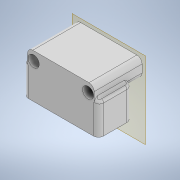
# Autodesk Inventor part: Кронштейн АКБ
Saved by Autodesk Inventor 2021 (Build 250183000, 183)
## iProperties
Created: 2023-02-18
Part Number: Кронштейн АКБ
Material: Типовые
Document SubType Name: Modeling
Designer: Tasya
Density: 1 g/cm^3
Appearance: По умолчанию
Author: Tasya
Autodesk Inventor part; units mm, degrees
ref_plane "YZ Plane" through (0, 0, 0) normal (1, 0, 0) x (0, 1, 0)
ref_plane "XZ Plane" through (0, 0, 0) normal (0, 1, 0) x (-1, 0, 0)
ref_plane "XY Plane" through (0, 0, 0) normal (0, 0, 1) x (1, 0, 0)
ref_plane "РабПлоскость1" through (0, 1, 4) normal (0, 0, 1) x (1, 0, 0)
sketch "Эскиз1" plane through (0, 1, 4) normal (0, 0, 1) x (1, 0, 0)
  circle A0 centre (-10.5, 2.5) radius 1.55 projected
  line L0 (12.85, -4) -> (12.85, 4) projected
  arc A1 (12.85, 4) -> (10.85, 6) centre (10.85, 4) ccw projected
  line L1 (10.85, 6) -> (-10.85, 6) projected
  arc A2 (-10.85, 6) -> (-12.85, 4) centre (-10.85, 4) ccw projected
  line L2 (-12.85, 4) -> (-12.85, -4) projected
  arc A3 (-12.85, -4) -> (-10.85, -6) centre (-10.85, -4) ccw construction
  line L3 (-10.85, -6) -> (-5, -6) construction
  line L4 (-3, -8) -> (-5, -6) construction
  line L5 (-3, -8) -> (-3, -21) construction
  line L6 (-3, -21) -> (3, -21) construction
  line L7 (3, -21) -> (3, -8) construction
  line L8 (5, -6) -> (3, -8) construction
  line L9 (5, -6) -> (10.85, -6) construction
  arc A4 (10.85, -6) -> (12.85, -4) centre (10.85, -4) ccw construction
  circle A5 centre (10.5, 2.5) radius 1.55 projected
  arc A6 (-12.85, 1) -> (-10.85, -1) centre (-10.85, 1) ccw projected
  line L10 (-10.85, -1) -> (10.85, -1) projected
  arc A7 (10.85, -1) -> (12.85, 1) centre (10.85, 1) ccw projected
  point P0 (0, -1)
extrude "Выдавливание1" add sketch "Эскиз1" along normal blind 18.5 contours A0 | A7 L10 A6 L2 A2 L1 A1 L0 | A5
sketch "Эскиз2" plane through (-10.85, 0, 4) normal (0, -1, 0) x (1, 0, 0)
  line L0 (10.85, -4) -> (10.85, 28) construction
  line L1 (23.35, 16.5) -> (-1.65, 16.5)
  line L2 (-1.65, 16.5) -> (-1.65, 7.5)
  line L3 (-1.65, 7.5) -> (23.35, 7.5)
  line L4 (23.35, 7.5) -> (23.35, 16.5)
  line L5 (23.35, 16.5) -> (-1.65, 7.5) construction
  line L6 (-1.65, 16.5) -> (23.35, 7.5) construction
  line L7 (-3.65, 7.5) -> (-3.65, 16.5)
  line L8 (-1.65, 18.5) -> (23.35, 18.5)
  line L9 (25.35, 16.5) -> (25.35, 7.5)
  line L10 (23.35, 5.5) -> (-1.65, 5.5)
  arc A0 (-3.65, 7.5) -> (-1.65, 5.5) centre (-1.65, 7.5) ccw
  arc A1 (-1.65, 18.5) -> (-3.65, 16.5) centre (-1.65, 16.5) ccw
  arc A2 (25.35, 16.5) -> (23.35, 18.5) centre (23.35, 16.5) ccw
  arc A3 (23.35, 5.5) -> (25.35, 7.5) centre (23.35, 7.5) ccw
  point P0 (10.85, 12)
  dimension "d2" = 25
  dimension "d3" = 9
  dimension "d4" = 16
  dimension "d5" = 2
  dimension "d6" = 2
  constraints: 22 end point, 8 point on circle, 8 tangent, 4 centre point, 4 parallel, 3 equal radius, 3 midpoint, 2 perpendicular, 1 horizontal, 1 vertical, 3 other
  measures "d2" distance of L1.start L1.end
  measures "d3" distance of L1.end L2.end
  measures "d4" distance of L0.start point (10.85, 12)
  measures "d5" distance between parallel lines of L2 L7
  measures "d6" radius of A0
extrude "Выдавливание2" add sketch "Эскиз2" along normal blind 10
sketch "Эскиз3" plane through (-10.85, 0, 4) normal (0, 1, 0) x (1, 0, 0)
  point P0 (10.85, 4)
sketch "Эскиз4" plane through (-10.85, 0, 4) normal (0, 1, 0) x (1, 0, 0)
  line L0 (21.7, -5.5) -> (21.7, -7.5) projected
  line L1 (23.35, -7.5) -> (21.7, -7.5) construction
  line L2 (23.35, -16.5) -> (23.35, -7.5) construction
  line L3 (21.7, -16.5) -> (23.35, -16.5) construction
  line L4 (21.7, -16.5) -> (21.7, -18.5) projected
  line L5 (23.35, -18.5) -> (21.7, -18.5) projected
  arc A0 (23.35, -18.5) -> (25.35, -16.5) centre (23.35, -16.5) ccw projected
  line L6 (25.35, -7.5) -> (25.35, -16.5) projected
  arc A1 (25.35, -7.5) -> (23.35, -5.5) centre (23.35, -7.5) ccw projected
  line L7 (21.7, -5.5) -> (23.35, -5.5) projected
  line L8 (21.7, -18.5) -> (0, -18.5) projected
  line L9 (-2, -18.5) -> (0, -18.5) projected
  arc A2 (-3.65, -16.5) -> (-1.65, -18.5) centre (-1.65, -16.5) ccw projected
  line L10 (-3.65, -16.5) -> (-3.65, -7.5) projected
  arc A3 (-1.65, -5.5) -> (-3.65, -7.5) centre (-1.65, -7.5) ccw projected
  line L11 (-1.65, -5.5) -> (0, -5.5) projected
  line L12 (21.7, -5.5) -> (0, -5.5) projected
  line L13 (21.7, -5.5) -> (23.35, -5.5) projected
  line L14 (21.7, -18.5) -> (23.7, -18.5) projected
  point P0 (10.85, 4)
extrude "Выдавливание3" add sketch "Эскиз4" along normal blind 2
fillet "Сопряжение1" radius 1 8 edges at (14.033, 2, 10.2155) (14.033, 2, 21.7845) (14.5, 2, 16) (12.85, 2, 16) (-14.033, 2, 21.7845) (-14.033, 2, 10.2155) (-14.5, 2, 16) (-12.85, 2, 16)
sketch "Эскиз5" plane through (0, 1, 22.5) normal (0, 0, 1) x (1, 0, 0)
  circle A0 centre (-10.5, 2.5) radius 1.55 construction
  circle A1 centre (10.5, 2.5) radius 1.55 construction
  point P0 (0, -1)
  constraints: 2 coincident
hole "Отверстие1" at (10.5, 3.5, 22.5) at (-10.5, 3.5, 22.5) direction (0, 0, -1) diameter 2.4 end through all counterbore diameter 4.3 counterbore depth 13 clearance for "винты со шлицем и цилиндрической головкой  ГОСТ 12876-67" size "M2" standard "ГОСТ"
